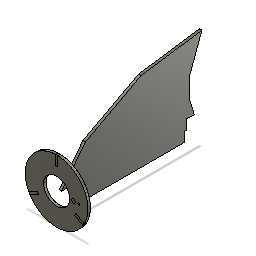
Babys First High Powered Rocket v7 (Autodesk Fusion 360 design; units mm, degrees)
Autodesk Fusion 360 part; units mm, degrees
note: some values were not read from the file. Set by a fixed rule: which sketch regions a step uses.
sketch "Sketch1" plane through (0, 0, 0) normal (1, 0, 0) x (0, 0, -1)
  line L0 (0, 0) -> (37.5, 48.4)
  line L1 (125, 95) -> (221, 109)
  line L2 (221, 109) -> (201, 55.1)
  line L3 (37.5, 48.4) -> (125, 95)
  line L4 (201, 55.1) -> (201, 25)
  line L5 (201, 25) -> (209, 0)
  line L6 (197, 0) -> (197, -15.1)
  line L7 (193.2, -30.2) -> (25.8, -30.2)
  line L8 (22, -15.1) -> (22, 0)
  line L9 (0, 0) -> (22, 0)
  line L10 (197, 0) -> (209, 0)
  line L11 (22, -15.1) -> (25.8, -15.1)
  line L12 (25.8, -15.1) -> (25.8, -30.2)
  line L13 (197, -15.1) -> (193.2, -15.1)
  line L14 (193.2, -15.1) -> (193.2, -30.2)
  dimension "d1" = 37.5
  dimension "d3" = 125
  dimension "d5" = 221
  dimension "d6" = 109
  dimension "d7" = 201
  dimension "d8" = 55.1
  dimension "d10" = 209
  dimension "d11" = 25
  dimension "d14" = 12
  dimension "d17" = 125.2
  dimension "d18" = 78.6
  dimension "d19" = 3.8
  dimension "d20" = 22
  dimension "d21" = 15.1
  dimension "d22" = 3.8
  dimension "d23" = 15.1
  dimension "d24" = 30.2
  dimension "d39" = 15.1
  constraint coincident L0.start L9.start
  constraint vertical L4
  constraint horizontal L9
  constraint coincident L6.start L9
  constraint perpendicular L6 L9
  constraint perpendicular L6 L7
  constraint perpendicular L8 L9
  constraint collinear L9 L10
  constraint perpendicular L8 L11
  constraint perpendicular L7 L12
  constraint perpendicular L6 L13
  constraint perpendicular L7 L14
  measures "d1" horizontal distance of L0.start L0.end
  measures "d3" horizontal distance of L0.start L1.start
  measures "d5" horizontal distance of L0.start L1.end
  measures "d6" vertical distance of L0.start L1.end
  measures "d7" horizontal distance of L0.start L2.end
  measures "d8" vertical distance of L0.start L2.end
  measures "d10" distance of L0.start L5.end
  measures "d11" vertical distance of L4.end L5.end
  measures "d14" distance of L5.end L6.start
  measures "d17" distance of L1.start L7
  measures "d18" distance of L0.end L7
  measures "d19" distance of L8.start L11.end
  measures "d20" distance of L0.start L8
  measures "d21" distance of L0.start L11
  measures "d22" distance of L6.end L13.end
  measures "d23" distance of L0.start L13
  measures "d24" distance of L0.start L7
  measures "d39" distance of L7 L8.start
extrude "Extrude1" add sketch "Sketch1" along normal blind 4 makes body 1
sketch "Sketch1 (2)" plane through (0, 0, 0) normal (0, 0, 1) x (1, 0, 0) in component "cr"
  circle A0 centre (0, 0) radius 20.525
  circle A1 centre (0, 0) radius 49.25
  circle A2 centre (35, 0) radius 1.75
  dimension "d25" = 41.05
  dimension "d26" = 98.5
  dimension "d44" = 35
  dimension "d45" = 3.5
  constraint coincident A0.centre A1.centre
  constraint concentric A0 A1
  constraint horizontal A0.centre A2.centre
  measures "d25" diameter of A0
  measures "d26" diameter of A1
  measures "d44" distance of A0.centre A2.centre
  measures "d45" diameter of A2
extrude "Extrude1'" add sketch "Sketch1 (2)" along normal blind 4 separate body makes body 2 in component "cr"
sketch "Sketch1 (3)" plane through (0, 0, 0) normal (0, 0, 1) x (1, 0, 0) in component "cr fin"
  circle A0 centre (0, 0) radius 20.525
  line L0 (-1.875, 34.15) -> (1.875, 34.15)
  line L1 (1.875, 34.15) -> (1.875, 49.2143)
  line L2 (-1.875, 34.15) -> (-1.875, 49.2143)
  line L3 (-28.6373, -18.6988) -> (-41.6833, -26.2309)
  line L4 (-30.5123, -15.4512) -> (-43.5583, -22.9834)
  line L5 (-28.6373, -18.6988) -> (-30.5123, -15.4512)
  line L6 (30.5123, -15.4512) -> (43.5583, -22.9834)
  line L7 (28.6373, -18.6988) -> (41.6833, -26.2309)
  line L8 (30.5123, -15.4512) -> (28.6373, -18.6988)
  arc A1 (-1.875, 49.2143) -> (-43.5583, -22.9834) centre (0, 0) ccw
  arc A2 (-41.6833, -26.2309) -> (41.6833, -26.2309) centre (0, 0) ccw
  arc A3 (43.5583, -22.9834) -> (1.875, 49.2143) centre (0, 0) ccw
  circle A4 centre (26.5, 0) radius 3
  line L9 (0, 0) -> (0, 34.15) construction
  line L10 (0, 20.525) -> (2.1631, 27.1824)
  line L11 (0, 20.525) -> (7, 20.525) construction
  line L12 (0, 20.525) -> (-2.1631, 27.1824)
  line L13 (0, 20.525) -> (7, 20.525) construction
  line L14 (-2.1631, 27.1824) -> (2.1631, 27.1824)
  line L15 (-17.7752, -10.2625) -> (-22.4591, -15.4645)
  line L16 (-22.4591, -15.4645) -> (-24.6222, -11.7179)
  line L17 (-17.7752, -10.2625) -> (-24.6222, -11.7179)
  line L18 (17.7752, -10.2625) -> (24.6222, -11.7179)
  line L19 (24.6222, -11.7179) -> (22.4591, -15.4645)
  line L20 (17.7752, -10.2625) -> (22.4591, -15.4645)
  dimension "d29" = 41.05
  dimension "d30" = 98.5
  dimension "d33" = 3.75
  dimension "d34" = 34.15
  dimension "d36" = 360
  dimension "d40" = 15.0643
  dimension "d48" = 6
  dimension "d49" = 26.5
  dimension "d51" = 72
  dimension "d52" = 7
  dimension "d53" = 108
  dimension "d54" = 7
  dimension "d56" = 360
  constraint coincident A0.centre A1.centre
  constraint perpendicular L0 L1
  constraint perpendicular L0 L2
  constraint concentric A1 A2
  constraint concentric A2 A3
  constraint horizontal A0.centre A4.centre
  constraint midpoint L0 L9.end
  constraint horizontal L11
  constraint coincident L9 L10.start
  constraint coincident A0 L10.start
  constraint horizontal L13
  measures "d29" diameter of A0
  measures "d30" diameter of A1
  measures "d33" distance of L0.start L0.end
  measures "d34" distance of A0.centre L0
  measures "d40" distance of L0.end L1.end
  measures "d48" diameter of A4
  measures "d49" distance of A0.centre A4.centre
  measures "d51" angle of L10 L11
  measures "d52" distance of L10.start L10.end
  measures "d53" angle of L12 L13
  measures "d54" distance of L10.start L12.end
extrude "Extrude2" add sketch "Sketch1 (3)" along normal blind 4 separate body contours L18 L19 L20 | L15 L16 L17 | L10 L12 L14 | L0 L1 L2 L3 L4 L5 L6 L7 L8 A1 A2 A3 | A4 makes body 3
extrude "Extrude3" cut sketch "Sketch1 (3)" along normal through all contours A4 bodies 3
extrude "Extrude4" cut sketch "Sketch1 (3)" along normal blind 0.1 contours L18 L19 L20 | L15 L16 L17 | L10 L12 L14 | L0 L1 L2 L3 L4 L5 L6 L7 L8 A1 A2 A3 bodies 3
extrude "Extrude5" cut sketch "Sketch1 (3)" along normal blind 0.15 contours L18 L19 L20 | L15 L16 L17 | L10 L12 L14 bodies 3
component "cr" placed x (1, 0, 0) y (0, 1, 0) z (0, 0, 1) at (0, 0, 0)
component "cr fin" placed x (1, 0, 0) y (0, 1, 0) z (0, 0, 1) at (0, 0, 0)
